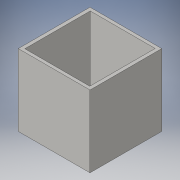
# Autodesk Inventor part: Part2
Saved by Autodesk Inventor 2016 (Build 200138000, 138)
## iProperties
Created: 2016-01-15
Part Number: Part2
Material: Generic
Document SubType Name: Modeling
Designer: Administrator
Density: 1 g/cm^3
Appearance: Default
Author: Administrator
Autodesk Inventor part; units mm, degrees
ref_plane "YZ Plane" through (0, 0, 0) normal (1, 0, 0) x (0, 1, 0)
ref_plane "XZ Plane" through (0, 0, 0) normal (0, 1, 0) x (-1, 0, 0)
ref_plane "XY Plane" through (0, 0, 0) normal (0, 0, 1) x (1, 0, 0)
sketch "Sketch1" plane through (0, 0, 0) normal (0, 1, 0) x (-1, 0, 0)
  line L0 (0, 0) -> (-50.8, 0)
  line L1 (-50.8, 0) -> (-50.8, 50.8)
  line L2 (-50.8, 50.8) -> (0, 50.8)
  line L3 (0, 50.8) -> (0, 0)
  dimension "d0" = 50.8
  dimension "d1" = 50.8
  constraints: 8 end point, 2 parallel, 1 horizontal, 1 perpendicular
  measures "d0" distance of L1.end L2.end
  measures "d1" distance of L0.end L1.end
extrude "Extrusion1" add sketch "Sketch1" along normal blind 50.8
sketch "Sketch2" plane through (0, 50.8, 0) normal (0, 1, 0) x (1, 0, 0)
  line L0 (2.4003, -48.5652) -> (48.3997, -48.5652)
  line L1 (48.3997, -48.5652) -> (48.3997, -2.2348)
  line L2 (48.3997, -2.2348) -> (2.4003, -2.2348)
  line L3 (2.4003, -2.2348) -> (2.4003, -48.5652)
  line L4 (2.4003, -48.5652) -> (48.3997, -2.2348) construction
  line L5 (48.3997, -48.5652) -> (2.4003, -2.2348) construction
  point P0 (0, 0)
  point P1 (25.4, -25.4)
  dimension "d4" = 45.9994
  constraints: 12 end point, 2 midpoint, 2 parallel, 1 horizontal, 1 perpendicular
  measures "d4" distance of L2.end L1.end
extrude "Extrusion2" cut sketch "Sketch2" against normal blind 50.8
body "Solid1"
